Autodesk Inventor part; units mm, degrees
(part 4 of 5)
  line L2308 (121.595, 74.0625) -> (121.595, 60.2629) projected
  line L2309 (121.595, 74.0625) -> (121.595, 60.2629) projected
  line L2310 (121.595, 60.2629) -> (107.794, 60.2629) projected
  line L2311 (121.595, 60.2629) -> (107.794, 60.2629) projected
  line L2312 (121.595, 74.0625) -> (121.595, 60.2629) projected
  line L2313 (121.595, 74.0625) -> (121.595, 60.2629) projected
  line L2314 (107.794, 74.0625) -> (121.595, 74.0625) projected
  line L2315 (107.794, 74.0625) -> (121.595, 74.0625) projected
  line L2316 (121.595, 60.2629) -> (107.794, 60.2629) projected
  line L2317 (121.595, 60.2629) -> (107.794, 60.2629) projected
  line L2318 (107.794, 60.2629) -> (107.794, 74.0625) projected
  line L2319 (107.794, 60.2629) -> (107.794, 74.0625) projected
  line L2320 (102.545, 74.0625) -> (102.545, 60.2629) projected
  line L2321 (102.545, 74.0625) -> (102.545, 60.2629) projected
  line L2322 (102.545, 60.2629) -> (88.7444, 60.2629) projected
  line L2323 (102.545, 60.2629) -> (88.7444, 60.2629) projected
  line L2324 (88.7444, 60.2629) -> (88.7444, 74.0625) projected
  line L2325 (88.7444, 60.2629) -> (88.7444, 74.0625) projected
  line L2326 (88.7444, 74.0625) -> (102.545, 74.0625) projected
  line L2327 (88.7444, 74.0625) -> (102.545, 74.0625) projected
  line L2328 (88.2579, 55.0125) -> (88.2579, 41.2129) projected
  line L2329 (88.2579, 55.0125) -> (88.2579, 41.2129) projected
  line L2330 (88.2579, 41.2129) -> (74.4583, 41.2129) projected
  line L2331 (88.2579, 41.2129) -> (74.4583, 41.2129) projected
  line L2332 (74.4583, 55.0125) -> (88.2579, 55.0125) projected
  line L2333 (74.4583, 55.0125) -> (88.2579, 55.0125) projected
  line L2334 (74.4583, 41.2129) -> (74.4583, 55.0125) projected
  line L2335 (74.4583, 41.2129) -> (74.4583, 55.0125) projected
  line L2336 (69.2079, 55.0125) -> (69.2079, 41.2129) projected
  line L2337 (69.2079, 55.0125) -> (69.2079, 41.2129) projected
  line L2338 (93.5083, 41.2129) -> (93.5083, 55.0125) projected
  line L2339 (93.5083, 41.2129) -> (93.5083, 55.0125) projected
  line L2340 (112.07, 116.926) -> (112.07, 103.125) projected
  line L2341 (112.07, 103.125) -> (98.2694, 103.125) projected
  line L2342 (112.07, 103.125) -> (98.2694, 103.125) projected
  line L2343 (98.2694, 103.125) -> (98.2694, 116.926) projected
  line L2344 (98.2694, 116.926) -> (112.07, 116.926) projected
  line L2345 (98.2694, 116.926) -> (112.07, 116.926) projected
  line L2346 (112.07, 116.926) -> (112.07, 103.125) projected
  line L2347 (135.883, 116.926) -> (135.883, 103.125) projected
  line L2348 (135.883, 116.926) -> (135.883, 103.125) projected
  line L2349 (135.883, 103.125) -> (122.083, 103.125) projected
  line L2350 (98.2694, 103.125) -> (98.2694, 116.926) projected
  line L2351 (135.883, 103.125) -> (122.083, 103.125) projected
  line L2352 (73.9704, 116.926) -> (73.9704, 103.125) projected
  line L2353 (73.9704, 116.926) -> (73.9704, 103.125) projected
  line L2354 (93.0204, 103.125) -> (79.2194, 103.125) projected
  line L2355 (93.0204, 103.125) -> (79.2194, 103.125) projected
  line L2356 (93.0204, 116.926) -> (93.0204, 103.125) projected
  line L2357 (93.0204, 116.926) -> (93.0204, 103.125) projected
  line L2358 (93.0204, 116.926) -> (93.0204, 103.125) projected
  line L2359 (93.0204, 116.926) -> (93.0204, 103.125) projected
  line L2360 (93.0204, 93.1125) -> (93.0204, 79.3129) projected
  line L2361 (93.0204, 93.1125) -> (93.0204, 79.3129) projected
  line L2362 (79.2194, 79.3129) -> (79.2194, 93.1125) projected
  line L2363 (79.2194, 79.3129) -> (79.2194, 93.1125) projected
  line L2364 (79.2194, 93.1125) -> (93.0204, 93.1125) projected
  line L2365 (79.2194, 93.1125) -> (93.0204, 93.1125) projected
  line L2366 (93.0204, 103.125) -> (79.2194, 103.125) projected
  line L2367 (93.0204, 103.125) -> (79.2194, 103.125) projected
  line L2368 (79.2194, 116.926) -> (93.0204, 116.926) projected
  line L2369 (79.2194, 116.926) -> (93.0204, 116.926) projected
  line L2370 (79.2194, 116.926) -> (93.0204, 116.926) projected
  line L2371 (79.2194, 116.926) -> (93.0204, 116.926) projected
  line L2372 (79.2194, 103.125) -> (79.2194, 116.926) projected
  line L2373 (79.2194, 103.125) -> (79.2194, 116.926) projected
  line L2374 (79.2194, 103.125) -> (79.2194, 116.926) projected
  line L2375 (79.2194, 103.125) -> (79.2194, 116.926) projected
  line L2376 (73.9704, 103.125) -> (60.1694, 103.125) projected
  line L2377 (73.9704, 103.125) -> (60.1694, 103.125) projected
  line L2378 (60.1694, 103.125) -> (60.1694, 116.926) projected
  line L2379 (60.1694, 103.125) -> (60.1694, 116.926) projected
  line L2380 (60.1694, 116.926) -> (73.9704, 116.926) projected
  line L2381 (60.1694, 116.926) -> (73.9704, 116.926) projected
  line L2382 (54.919, 103.125) -> (41.1208, 103.125) projected
  line L2383 (54.919, 103.125) -> (41.1208, 103.125) projected
  line L2384 (41.1208, 103.125) -> (41.1208, 116.926) projected
  line L2385 (41.1208, 103.125) -> (41.1208, 116.926) projected
  line L2386 (41.1208, 116.926) -> (54.919, 116.926) projected
  line L2387 (41.1208, 116.926) -> (54.919, 116.926) projected
  line L2388 (54.919, 116.926) -> (54.919, 103.125) projected
  line L2389 (73.9704, 103.125) -> (60.1694, 103.125) projected
  line L2390 (73.9704, 103.125) -> (60.1694, 103.125) projected
  line L2391 (60.1694, 116.926) -> (73.9704, 116.926) projected
  line L2392 (60.1694, 116.926) -> (73.9704, 116.926) projected
  line L2393 (73.9704, 116.926) -> (73.9704, 103.125) projected
  line L2394 (73.9704, 116.926) -> (73.9704, 103.125) projected
  line L2395 (41.1208, 93.1125) -> (54.919, 93.1125) projected
  line L2396 (41.1208, 93.1125) -> (54.919, 93.1125) projected
  line L2397 (41.1208, 93.1125) -> (54.919, 93.1125) projected
  line L2398 (60.1694, 103.125) -> (60.1694, 116.926) projected
  line L2399 (60.1694, 103.125) -> (60.1694, 116.926) projected
  line L2400 (54.919, 103.125) -> (41.1208, 103.125) projected
  line L2401 (54.919, 103.125) -> (41.1208, 103.125) projected
  line L2402 (54.919, 116.926) -> (54.919, 103.125) projected
  line L2403 (54.919, 116.926) -> (54.919, 103.125) projected
  line L2404 (54.919, 116.926) -> (54.919, 103.125) projected
  line L2405 (41.1208, 116.926) -> (54.919, 116.926) projected
  line L2406 (41.1208, 116.926) -> (54.919, 116.926) projected
  line L2407 (41.1208, 93.1125) -> (54.919, 93.1125) projected
  line L2408 (88.7444, 60.2629) -> (88.7444, 74.0625) projected
  line L2409 (88.7444, 60.2629) -> (88.7444, 74.0625) projected
  line L2410 (79.2194, 79.3129) -> (79.2194, 93.1125) projected
  line L2411 (79.2194, 79.3129) -> (79.2194, 93.1125) projected
  line L2412 (79.2194, 93.1125) -> (93.0204, 93.1125) projected
  line L2413 (79.2194, 93.1125) -> (93.0204, 93.1125) projected
  line L2414 (93.0204, 93.1125) -> (93.0204, 79.3129) projected
  line L2415 (93.0204, 93.1125) -> (93.0204, 79.3129) projected
  line L2416 (93.0204, 79.3129) -> (79.2194, 79.3129) projected
  line L2417 (93.0204, 79.3129) -> (79.2194, 79.3129) projected
  line L2418 (83.4954, 60.2629) -> (69.6958, 60.2629) projected
  line L2419 (69.6958, 74.0625) -> (83.4954, 74.0625) projected
  line L2420 (69.6958, 74.0625) -> (83.4954, 74.0625) projected
  line L2421 (83.4954, 74.0625) -> (83.4954, 60.2629) projected
  line L2422 (83.4954, 74.0625) -> (83.4954, 60.2629) projected
  line L2423 (83.4954, 60.2629) -> (69.6958, 60.2629) projected
  line L2424 (83.4954, 60.2629) -> (69.6958, 60.2629) projected
  line L2425 (83.4954, 74.0625) -> (83.4954, 60.2629) projected
  line L2426 (83.4954, 74.0625) -> (83.4954, 60.2629) projected
  line L2427 (69.6958, 74.0625) -> (83.4954, 74.0625) projected
  line L2428 (69.6958, 74.0625) -> (83.4954, 74.0625) projected
  line L2429 (93.0204, 79.3129) -> (79.2194, 79.3129) projected
  line L2430 (93.0204, 79.3129) -> (79.2194, 79.3129) projected
  line L2431 (83.4954, 60.2629) -> (69.6958, 60.2629) projected
  line L2432 (41.1208, 79.3129) -> (41.1208, 93.1125) projected
  line L2433 (41.1208, 79.3129) -> (41.1208, 93.1125) projected
  line L2434 (16.8203, 103.125) -> (3.0193, 103.125) projected
  line L2435 (16.8203, 103.125) -> (3.0193, 103.125) projected
  line L2436 (3.0193, 103.125) -> (3.0193, 116.926) projected
  line L2437 (3.0193, 103.125) -> (3.0193, 116.926) projected
  line L2438 (3.0193, 116.926) -> (16.8203, 116.926) projected
  line L2439 (3.0193, 116.926) -> (16.8203, 116.926) projected
  line L2440 (3.0193, 79.3129) -> (3.0193, 93.1125) projected
  line L2441 (3.0193, 93.1125) -> (16.8203, 93.1125) projected
  line L2442 (3.0193, 93.1125) -> (16.8203, 93.1125) projected
  line L2443 (16.8203, 93.1125) -> (16.8203, 79.3129) projected
  line L2444 (16.8203, 93.1125) -> (16.8203, 79.3129) projected
  line L2445 (16.8203, 93.1125) -> (16.8203, 79.3129) projected
  line L2446 (16.8203, 93.1125) -> (16.8203, 79.3129) projected
  line L2447 (3.0193, 93.1125) -> (16.8203, 93.1125) projected
  line L2448 (3.0193, 93.1125) -> (16.8203, 93.1125) projected
  line L2449 (3.0193, 79.3129) -> (3.0193, 93.1125) projected
  line L2450 (3.0193, 79.3129) -> (3.0193, 93.1125) projected
  line L2451 (22.0707, 79.3129) -> (22.0707, 93.1125) projected
  line L2452 (22.0707, 79.3129) -> (22.0707, 93.1125) projected
  line L2453 (0.0951, 117.85) -> (0.0951, 2.1869) projected
  line L2454 (0.0951, 117.85) -> (0.0951, 2.187) projected
  line L2455 (41.1208, 103.125) -> (41.1208, 116.926) projected
  line L2456 (41.1208, 103.125) -> (41.1208, 116.926) projected
  line L2457 (16.8203, 116.926) -> (16.8203, 103.125) projected
  line L2458 (16.8203, 116.926) -> (16.8203, 103.125) projected
  line L2459 (3.0193, 79.3129) -> (3.0193, 93.1125) projected
  line L2460 (22.0707, 79.3129) -> (22.0707, 93.1125) projected
  line L2461 (22.0707, 79.3129) -> (22.0707, 93.1125) projected
  line L2462 (35.8704, 79.3129) -> (22.0707, 79.3129) projected
  line L2463 (35.8704, 79.3129) -> (22.0707, 79.3129) projected
  line L2464 (35.8704, 79.3129) -> (22.0707, 79.3129) projected
  line L2465 (22.0707, 93.1125) -> (35.8704, 93.1125) projected
  line L2466 (22.0707, 93.1125) -> (35.8704, 93.1125) projected
  line L2467 (22.0707, 93.1125) -> (35.8704, 93.1125) projected
  line L2468 (35.8704, 79.3129) -> (22.0707, 79.3129) projected
  line L2469 (22.0707, 93.1125) -> (35.8704, 93.1125) projected
  line L2470 (35.8704, 93.1125) -> (35.8704, 79.3129) projected
  line L2471 (35.8704, 93.1125) -> (35.8704, 79.3129) projected
  line L2472 (35.8704, 93.1125) -> (35.8704, 79.3129) projected
  line L2473 (35.8704, 93.1125) -> (35.8704, 79.3129) projected
  line L2474 (31.5957, 60.2629) -> (31.5957, 74.0625) projected
  line L2475 (31.5957, 60.2629) -> (31.5957, 74.0625) projected
  line L2476 (31.5957, 60.2629) -> (31.5957, 74.0625) projected
  line L2477 (31.5957, 74.0625) -> (45.3954, 74.0625) projected
  line L2478 (31.5957, 74.0625) -> (45.3954, 74.0625) projected
  line L2479 (31.5957, 74.0625) -> (45.3954, 74.0625) projected
  line L2480 (31.5957, 74.0625) -> (45.3954, 74.0625) projected
  line L2481 (31.5957, 60.2629) -> (31.5957, 74.0625) projected
  line L2482 (16.8203, 79.3129) -> (3.0193, 79.3129) projected
  line L2483 (16.8203, 79.3129) -> (3.0193, 79.3129) projected
  line L2484 (7.7832, 74.0625) -> (21.5828, 74.0625) projected
  line L2485 (7.7832, 74.0625) -> (21.5828, 74.0625) projected
  line L2486 (21.5828, 74.0625) -> (21.5828, 60.2629) projected
  line L2487 (21.5828, 74.0625) -> (21.5828, 60.2629) projected
  line L2488 (7.7832, 60.2629) -> (7.7832, 74.0625) projected
  line L2489 (7.7832, 60.2629) -> (7.7832, 74.0625) projected
  line L2490 (7.7832, 60.2629) -> (7.7832, 74.0625) projected
  line L2491 (7.7832, 60.2629) -> (7.7832, 74.0625) projected
  line L2492 (21.5828, 74.0625) -> (21.5828, 60.2629) projected
  line L2493 (21.5828, 74.0625) -> (21.5828, 60.2629) projected
  line L2494 (16.8203, 79.3129) -> (3.0193, 79.3129) projected
  line L2495 (16.8203, 79.3129) -> (3.0193, 79.3129) projected
  line L2496 (21.5828, 60.2629) -> (7.7832, 60.2629) projected
  line L2497 (21.5828, 60.2629) -> (7.7832, 60.2629) projected
  line L2498 (21.5828, 60.2629) -> (7.7832, 60.2629) projected
  line L2499 (21.5828, 60.2629) -> (7.7832, 60.2629) projected
  line L2500 (10.163, 55.0125) -> (23.9641, 55.0125) projected
  line L2501 (10.163, 55.0125) -> (23.9641, 55.0125) projected
  line L2502 (10.163, 55.0125) -> (23.9641, 55.0125) projected
  line L2503 (10.163, 55.0125) -> (23.9641, 55.0125) projected
  line L2504 (23.9641, 55.0125) -> (23.9641, 41.2129) projected
  line L2505 (23.9641, 55.0125) -> (23.9641, 41.2129) projected
  line L2506 (23.9641, 55.0125) -> (23.9641, 41.2129) projected
  line L2507 (23.9641, 55.0125) -> (23.9641, 41.2129) projected
  line L2508 (10.163, 41.2129) -> (10.163, 55.0125) projected
  line L2509 (10.163, 41.2129) -> (10.163, 55.0125) projected
  line L2510 (10.163, 41.2129) -> (10.163, 55.0125) projected
  line L2511 (10.163, 41.2129) -> (10.163, 55.0125) projected
  line L2512 (23.9641, 41.2129) -> (10.163, 41.2129) projected
  line L2513 (23.9641, 41.2129) -> (10.163, 41.2129) projected
  line L2514 (23.9641, 41.2129) -> (10.163, 41.2129) projected
  line L2515 (23.9641, 41.2129) -> (10.163, 41.2129) projected
  line L2516 (45.3954, 60.2629) -> (31.5957, 60.2629) projected
  line L2517 (45.3954, 60.2629) -> (31.5957, 60.2629) projected
  line L2518 (50.1579, 55.0125) -> (50.1579, 41.2129) projected
  line L2519 (50.1579, 55.0125) -> (50.1579, 41.2129) projected
  line L2520 (45.8833, 35.9625) -> (59.6829, 35.9625) projected
  line L2521 (45.8833, 35.9625) -> (59.6829, 35.9625) projected
  line L2522 (50.1579, 55.0125) -> (50.1579, 41.2129) projected
  line L2523 (50.1579, 55.0125) -> (50.1579, 41.2129) projected
  line L2524 (37.0018, 31.2636) -> (37.8273, 31.2636) projected
  line L2525 (37.0018, 31.2636) -> (37.8273, 31.2636) projected
  line L2526 (37.0018, 34.4923) -> (37.0018, 31.2636) projected
  line L2527 (37.0018, 34.4923) -> (37.0018, 31.2636) projected
  line L2528 (50.1579, 41.2129) -> (36.3583, 41.2129) projected
  line L2529 (50.1579, 41.2129) -> (36.3583, 41.2129) projected
  line L2530 (50.1579, 41.2129) -> (36.3583, 41.2129) projected
  line L2531 (50.1579, 41.2129) -> (36.3583, 41.2129) projected
  line L2532 (36.3583, 55.0125) -> (50.1579, 55.0125) projected
  line L2533 (36.3583, 55.0125) -> (50.1579, 55.0125) projected
  line L2534 (36.3583, 55.0125) -> (50.1579, 55.0125) projected
  line L2535 (36.3583, 55.0125) -> (50.1579, 55.0125) projected
  line L2536 (36.3583, 41.2129) -> (36.3583, 55.0125) projected
  line L2537 (36.3583, 41.2129) -> (36.3583, 55.0125) projected
  line L2538 (36.3583, 41.2129) -> (36.3583, 55.0125) projected
  line L2539 (36.3583, 41.2129) -> (36.3583, 55.0125) projected
  line L2540 (45.3954, 60.2629) -> (31.5957, 60.2629) projected
  line L2541 (45.3954, 60.2629) -> (31.5957, 60.2629) projected
  line L2542 (84.6391, 7.8135) -> (84.6391, 3.3431) projected
  line L2543 (84.6391, 7.8135) -> (84.6391, 3.3431) projected
  line L2544 (84.6391, 3.3431) -> (82.9137, 3.3431) projected
  line L2545 (84.6391, 3.3431) -> (82.9137, 3.3431) projected
  line L2546 (82.9137, 3.3431) -> (82.9137, 2.1429) projected
  line L2547 (82.9137, 3.3431) -> (82.9137, 2.1429) projected
  line L2548 (82.9137, 2.1429) -> (79.8132, 2.1429) projected
  line L2549 (82.9137, 2.1429) -> (79.8132, 2.1429) projected
  line L2550 (79.8132, 2.1429) -> (79.8132, 3.3431) projected
  line L2551 (78.0881, 3.3431) -> (78.0881, 9.6132) projected
  line L2552 (78.0881, 3.3431) -> (78.0881, 9.6132) projected
  line L2553 (78.0881, 3.3431) -> (78.0881, 9.6132) projected
  line L2554 (78.0881, 3.3431) -> (78.0881, 9.6132) projected
  line L2555 (84.6391, 7.8135) -> (84.6391, 3.3431) projected
  line L2556 (84.6391, 7.8135) -> (84.6391, 3.3431) projected
  line L2557 (84.6391, 3.3431) -> (82.9137, 3.3431) projected
  line L2558 (84.6391, 3.3431) -> (82.9137, 3.3431) projected
  line L2559 (79.8132, 3.3431) -> (78.0881, 3.3431) projected
  line L2560 (79.8132, 3.3431) -> (78.0881, 3.3431) projected
  line L2561 (79.8132, 3.3431) -> (78.0881, 3.3431) projected
  line L2562 (79.8132, 3.3431) -> (78.0881, 3.3431) projected
  line L2563 (79.8132, 2.1429) -> (79.8132, 3.3431) projected
  line L2564 (79.8132, 2.1429) -> (79.8132, 3.3431) projected
  line L2565 (79.8132, 2.1429) -> (79.8132, 3.3431) projected
  line L2566 (82.9137, 3.3431) -> (82.9137, 2.1429) projected
  line L2567 (82.9137, 3.3431) -> (82.9137, 2.1429) projected
  line L2568 (82.9137, 2.1429) -> (79.8132, 2.1429) projected
  line L2569 (82.9137, 2.1429) -> (79.8132, 2.1429) projected
  line L2570 (28.7266, 35.9625) -> (28.7266, 31.2636) projected
  line L2571 (28.7266, 35.9625) -> (28.7266, 31.2636) projected
  line L2572 (28.7266, 31.2636) -> (30.4519, 31.2636) projected
  line L2573 (28.7266, 26.8635) -> (28.7266, 22.163) projected
  line L2574 (28.7266, 26.8635) -> (28.7266, 22.163) projected
  line L2575 (30.4519, 26.8635) -> (28.7266, 26.8635) projected
  line L2576 (30.4519, 26.8635) -> (28.7266, 26.8635) projected
  line L2577 (30.4519, 26.8635) -> (28.7266, 26.8635) projected
  line L2578 (30.4519, 26.8635) -> (28.7266, 26.8635) projected
  line L2579 (30.4519, 22.3931) -> (30.4519, 26.8635) projected
  line L2580 (30.4519, 22.3931) -> (30.4519, 26.8635) projected
  line L2581 (32.1758, 21.1928) -> (32.1758, 22.3931) projected
  line L2582 (32.1758, 21.1928) -> (32.1758, 22.3931) projected
  line L2583 (32.1758, 22.3931) -> (30.4519, 22.3931) projected
  line L2584 (32.1758, 22.3931) -> (30.4519, 22.3931) projected
  line L2585 (28.7266, 31.2636) -> (30.4519, 31.2636) projected
  line L2586 (28.7266, 31.2636) -> (30.4519, 31.2636) projected
  line L2587 (28.7266, 31.2636) -> (30.4519, 31.2636) projected
  line L2588 (28.7266, 35.9625) -> (28.7266, 31.2636) projected
  line L2589 (28.7266, 35.9625) -> (28.7266, 31.2636) projected
  line L2590 (30.4519, 31.2636) -> (30.4519, 34.4923) projected
  line L2591 (30.4519, 31.2636) -> (30.4519, 34.4923) projected
  line L2592 (30.4519, 31.2636) -> (30.4519, 34.4923) projected
  line L2593 (30.4519, 31.2636) -> (30.4519, 34.4923) projected
  line L2594 (30.4519, 34.4923) -> (37.0018, 34.4923) projected
  line L2595 (30.4519, 34.4923) -> (37.0018, 34.4923) projected
  line L2596 (30.4519, 34.4923) -> (37.0018, 34.4923) projected
  line L2597 (30.4519, 34.4923) -> (37.0018, 34.4923) projected
  line L2598 (28.7266, 26.8635) -> (28.7266, 22.163) projected
  line L2599 (28.7266, 26.8635) -> (28.7266, 22.163) projected
  line L2600 (14.9269, 31.2636) -> (14.9269, 35.9625) projected
  line L2601 (14.9269, 31.2636) -> (14.9269, 35.9625) projected
  line L2602 (14.9269, 31.2636) -> (14.9269, 35.9625) projected
  line L2603 (14.9269, 31.2636) -> (14.9269, 35.9625) projected
  line L2604 (37.0018, 34.4923) -> (37.0018, 31.2636) projected
  line L2605 (37.0018, 34.4923) -> (37.0018, 31.2636) projected
  line L2606 (37.0018, 28.6632) -> (37.0018, 22.3931) projected
  line L2607 (37.0018, 28.6632) -> (37.0018, 22.3931) projected
  line L2608 (37.0018, 28.6632) -> (37.0018, 22.3931) projected
  line L2609 (37.0018, 28.6632) -> (37.0018, 22.3931) projected
  line L2610 (37.8273, 28.6632) -> (37.0018, 28.6632) projected
  line L2611 (37.8273, 28.6632) -> (37.0018, 28.6632) projected
  line L2612 (37.8273, 28.6632) -> (37.0018, 28.6632) projected
  line L2613 (37.8273, 28.6632) -> (37.0018, 28.6632) projected
  line L2614 (37.0018, 31.2636) -> (37.8273, 31.2636) projected
  line L2615 (37.0018, 31.2636) -> (37.8273, 31.2636) projected
  line L2616 (37.8273, 31.2636) -> (37.8273, 28.6632) projected
  line L2617 (37.8273, 31.2636) -> (37.8273, 28.6632) projected
  line L2618 (45.8833, 22.163) -> (45.8833, 35.9625) projected
  line L2619 (45.8833, 22.163) -> (45.8833, 35.9625) projected
  line L2620 (59.6829, 22.163) -> (45.8833, 22.163) projected
  line L2621 (59.6829, 22.163) -> (45.8833, 22.163) projected
  line L2622 (59.6829, 35.9625) -> (59.6829, 22.163) projected
  line L2623 (59.6829, 35.9625) -> (59.6829, 22.163) projected
  line L2624 (37.8273, 31.2636) -> (37.8273, 28.6632) projected
  line L2625 (37.8273, 31.2636) -> (37.8273, 28.6632) projected
  line L2626 (32.1758, 22.3931) -> (30.4519, 22.3931) projected
  line L2627 (32.1758, 22.3931) -> (30.4519, 22.3931) projected
  line L2628 (30.4519, 22.3931) -> (30.4519, 26.8635) projected
  line L2629 (30.4519, 22.3931) -> (30.4519, 26.8635) projected
  line L2630 (37.0018, 22.3931) -> (35.2764, 22.3931) projected
  line L2631 (37.0018, 22.3931) -> (35.2764, 22.3931) projected
  line L2632 (37.0018, 22.3931) -> (35.2764, 22.3931) projected
  line L2633 (37.0018, 22.3931) -> (35.2764, 22.3931) projected
  line L2634 (35.2764, 22.3931) -> (35.2764, 21.1928) projected
  line L2635 (35.2764, 22.3931) -> (35.2764, 21.1928) projected
  line L2636 (35.2764, 22.3931) -> (35.2764, 21.1928) projected
  line L2637 (35.2764, 22.3931) -> (35.2764, 21.1928) projected
  line L2638 (35.2764, 21.1928) -> (32.1758, 21.1928) projected
  line L2639 (35.2764, 21.1928) -> (32.1758, 21.1928) projected
  line L2640 (35.2764, 21.1928) -> (32.1758, 21.1928) projected
  line L2641 (35.2764, 21.1928) -> (32.1758, 21.1928) projected
  line L2642 (32.1758, 21.1928) -> (32.1758, 22.3931) projected
  line L2643 (32.1758, 21.1928) -> (32.1758, 22.3931) projected
  line L2644 (29.213, 16.9127) -> (43.0142, 16.9127) projected
  line L2645 (29.213, 16.9127) -> (43.0142, 16.9127) projected
  line L2646 (43.0142, 16.9127) -> (43.0142, 3.113) projected
  line L2647 (43.0142, 16.9127) -> (43.0142, 3.113) projected
  line L2648 (29.213, 3.113) -> (29.213, 16.9127) projected
  line L2649 (29.213, 3.113) -> (29.213, 16.9127) projected
  line L2650 (43.0142, 3.113) -> (29.213, 3.113) projected
  line L2651 (43.0142, 3.113) -> (29.213, 3.113) projected
  line L2652 (74.4583, 41.2129) -> (74.4583, 55.0125) projected
  line L2653 (74.4583, 41.2129) -> (74.4583, 55.0125) projected
  line L2654 (74.4583, 55.0125) -> (88.2579, 55.0125) projected
  line L2655 (74.4583, 55.0125) -> (88.2579, 55.0125) projected
  line L2656 (88.2579, 55.0125) -> (88.2579, 41.2129) projected
  line L2657 (88.2579, 55.0125) -> (88.2579, 41.2129) projected
  line L2658 (88.2579, 41.2129) -> (74.4583, 41.2129) projected
  line L2659 (88.2579, 41.2129) -> (74.4583, 41.2129) projected
  line L2660 (83.9833, 22.163) -> (83.9833, 35.9625) projected
  line L2661 (83.9833, 22.163) -> (83.9833, 35.9625) projected
  line L2662 (78.7329, 22.163) -> (64.9333, 22.163) projected
  line L2663 (78.7329, 22.163) -> (64.9333, 22.163) projected
  line L2664 (64.9333, 22.163) -> (64.9333, 35.9625) projected
  line L2665 (64.9333, 22.163) -> (64.9333, 35.9625) projected
  line L2666 (64.9333, 35.9625) -> (78.7329, 35.9625) projected
  line L2667 (64.9333, 35.9625) -> (78.7329, 35.9625) projected
  line L2668 (78.7329, 35.9625) -> (78.7329, 22.163) projected
  line L2669 (78.7329, 35.9625) -> (78.7329, 22.163) projected
  line L2670 (78.7329, 22.163) -> (64.9333, 22.163) projected
  line L2671 (78.7329, 22.163) -> (64.9333, 22.163) projected
  line L2672 (64.9333, 35.9625) -> (78.7329, 35.9625) projected
  line L2673 (64.9333, 35.9625) -> (78.7329, 35.9625) projected
  line L2674 (64.9333, 22.163) -> (64.9333, 35.9625) projected
  line L2675 (64.9333, 22.163) -> (64.9333, 35.9625) projected
  line L2676 (55.4083, 41.2129) -> (55.4083, 55.0125) projected
  line L2677 (55.4083, 41.2129) -> (55.4083, 55.0125) projected
  line L2678 (55.4083, 41.2129) -> (55.4083, 55.0125) projected
  line L2679 (55.4083, 41.2129) -> (55.4083, 55.0125) projected
  line L2680 (55.4083, 55.0125) -> (69.2079, 55.0125) projected
  line L2681 (55.4083, 55.0125) -> (69.2079, 55.0125) projected
  line L2682 (69.2079, 55.0125) -> (69.2079, 41.2129) projected
  line L2683 (69.2079, 55.0125) -> (69.2079, 41.2129) projected
  line L2684 (55.4083, 55.0125) -> (69.2079, 55.0125) projected
  line L2685 (55.4083, 55.0125) -> (69.2079, 55.0125) projected
  line L2686 (69.2079, 41.2129) -> (55.4083, 41.2129) projected
  line L2687 (69.2079, 41.2129) -> (55.4083, 41.2129) projected
  line L2688 (69.2079, 41.2129) -> (55.4083, 41.2129) projected
  line L2689 (69.2079, 41.2129) -> (55.4083, 41.2129) projected
  line L2690 (13.2016, 31.2636) -> (14.9269, 31.2636) projected
  line L2691 (13.2016, 31.2636) -> (14.9269, 31.2636) projected
  line L2692 (13.2016, 31.2636) -> (14.9269, 31.2636) projected
  line L2693 (13.2016, 31.2636) -> (14.9269, 31.2636) projected
  line L2694 (5.8263, 28.6632) -> (5.8263, 31.2636) projected
  line L2695 (5.8263, 28.6632) -> (5.8263, 31.2636) projected
  line L2696 (5.8263, 28.6632) -> (5.8263, 31.2636) projected
  line L2697 (5.8263, 28.6632) -> (5.8263, 31.2636) projected
  line L2698 (5.8263, 31.2636) -> (6.6518, 31.2636) projected
  line L2699 (5.8263, 31.2636) -> (6.6518, 31.2636) projected
  line L2700 (5.8263, 31.2636) -> (6.6518, 31.2636) projected
  line L2701 (6.6518, 34.4923) -> (13.2016, 34.4923) projected
  line L2702 (13.2016, 34.4923) -> (13.2016, 31.2636) projected
  line L2703 (13.2016, 34.4923) -> (13.2016, 31.2636) projected
  line L2704 (13.2016, 34.4923) -> (13.2016, 31.2636) projected
  line L2705 (6.6518, 34.4923) -> (13.2016, 34.4923) projected
  line L2706 (6.6518, 34.4923) -> (13.2016, 34.4923) projected
  line L2707 (6.6518, 34.4923) -> (13.2016, 34.4923) projected
  line L2708 (13.2016, 34.4923) -> (13.2016, 31.2636) projected
  line L2709 (6.6518, 31.2636) -> (6.6518, 34.4923) projected
  line L2710 (6.6518, 31.2636) -> (6.6518, 34.4923) projected
  line L2711 (6.6518, 31.2636) -> (6.6518, 34.4923) projected
  line L2712 (6.6518, 31.2636) -> (6.6518, 34.4923) projected
  line L2713 (5.8263, 31.2636) -> (6.6518, 31.2636) projected
  line L2714 (13.2016, 22.3931) -> (11.4763, 22.3931) projected
  line L2715 (13.2016, 22.3931) -> (11.4763, 22.3931) projected
  line L2716 (11.4763, 22.3931) -> (11.4763, 21.1928) projected
  line L2717 (11.4763, 22.3931) -> (11.4763, 21.1928) projected
  line L2718 (11.4763, 21.1928) -> (8.3771, 21.1928) projected
  line L2719 (11.4763, 21.1928) -> (8.3771, 21.1928) projected
  line L2720 (8.3771, 21.1928) -> (8.3771, 22.3931) projected
  line L2721 (8.3771, 21.1928) -> (8.3771, 22.3931) projected
  line L2722 (8.3771, 22.3931) -> (6.6518, 22.3931) projected
  line L2723 (8.3771, 22.3931) -> (6.6518, 22.3931) projected
  line L2724 (11.4763, 22.3931) -> (11.4763, 21.1928) projected
  line L2725 (11.4763, 22.3931) -> (11.4763, 21.1928) projected
  line L2726 (11.4763, 21.1928) -> (8.3771, 21.1928) projected
  line L2727 (11.4763, 21.1928) -> (8.3771, 21.1928) projected
  line L2728 (8.3771, 21.1928) -> (8.3771, 22.3931) projected
  line L2729 (8.3771, 21.1928) -> (8.3771, 22.3931) projected
  line L2730 (5.4019, 16.9127) -> (19.2016, 16.9127) projected
  line L2731 (5.4019, 16.9127) -> (19.2016, 16.9127) projected
  line L2732 (5.4019, 3.113) -> (5.4019, 16.9127) projected
  line L2733 (5.4019, 3.113) -> (5.4019, 16.9127) projected
  line L2734 (19.2016, 3.113) -> (5.4019, 3.113) projected
  line L2735 (19.2016, 3.113) -> (5.4019, 3.113) projected
  line L2736 (19.2016, 16.9127) -> (19.2016, 3.113) projected
  line L2737 (19.2016, 16.9127) -> (19.2016, 3.113) projected
  line L2738 (13.2016, 22.3931) -> (11.4763, 22.3931) projected
  line L2739 (13.2016, 22.3931) -> (11.4763, 22.3931) projected
  line L2740 (78.0881, 15.4423) -> (84.6391, 15.4423) projected
  line L2741 (78.0881, 15.4423) -> (84.6391, 15.4423) projected
  line L2742 (84.6391, 15.4423) -> (84.6391, 12.2136) projected
  line L2743 (84.6391, 15.4423) -> (84.6391, 12.2136) projected
  line L2744 (78.0881, 9.6132) -> (77.264, 9.6132) projected
  line L2745 (78.0881, 9.6132) -> (77.264, 9.6132) projected
  line L2746 (78.0881, 9.6132) -> (77.264, 9.6132) projected
  line L2747 (78.0881, 9.6132) -> (77.264, 9.6132) projected
  line L2748 (77.264, 12.2136) -> (78.0881, 12.2136) projected
  line L2749 (77.264, 9.6132) -> (77.264, 12.2136) projected
  line L2750 (77.264, 9.6132) -> (77.264, 12.2136) projected
  line L2751 (77.264, 9.6132) -> (77.264, 12.2136) projected
  line L2752 (77.264, 12.2136) -> (78.0881, 12.2136) projected
  line L2753 (77.264, 12.2136) -> (78.0881, 12.2136) projected
  line L2754 (77.264, 12.2136) -> (78.0881, 12.2136) projected
  line L2755 (84.6391, 15.4423) -> (84.6391, 12.2136) projected
  line L2756 (84.6391, 15.4423) -> (84.6391, 12.2136) projected
  line L2757 (78.0881, 15.4423) -> (84.6391, 15.4423) projected
  line L2758 (78.0881, 15.4423) -> (84.6391, 15.4423) projected
  line L2759 (78.0881, 12.2136) -> (78.0881, 15.4423) projected
  line L2760 (78.0881, 12.2136) -> (78.0881, 15.4423) projected
  line L2761 (78.0881, 12.2136) -> (78.0881, 15.4423) projected
  line L2762 (78.0881, 12.2136) -> (78.0881, 15.4423) projected
  line L2763 (77.264, 9.6132) -> (77.264, 12.2136) projected
  line L2764 (69.6958, 60.2629) -> (69.6958, 74.0625) projected
  line L2765 (69.6958, 60.2629) -> (69.6958, 74.0625) projected
  line L2766 (64.4454, 74.0625) -> (64.4454, 60.2629) projected
  line L2767 (64.4454, 74.0625) -> (64.4454, 60.2629) projected
  line L2768 (64.4454, 74.0625) -> (64.4454, 60.2629) projected
  line L2769 (64.4454, 74.0625) -> (64.4454, 60.2629) projected
  line L2770 (64.4454, 60.2629) -> (50.6458, 60.2629) projected
  line L2771 (64.4454, 60.2629) -> (50.6458, 60.2629) projected
  line L2772 (64.4454, 60.2629) -> (50.6458, 60.2629) projected
  line L2773 (64.4454, 60.2629) -> (50.6458, 60.2629) projected
  line L2774 (50.6458, 74.0625) -> (64.4454, 74.0625) projected
  line L2775 (50.6458, 60.2629) -> (50.6458, 74.0625) projected
  line L2776 (50.6458, 74.0625) -> (64.4454, 74.0625) projected
  line L2777 (50.6458, 60.2629) -> (50.6458, 74.0625) projected
  line L2778 (50.6458, 60.2629) -> (50.6458, 74.0625) projected
  line L2779 (50.6458, 60.2629) -> (50.6458, 74.0625) projected
  line L2780 (50.6458, 74.0625) -> (64.4454, 74.0625) projected
  line L2781 (50.6458, 74.0625) -> (64.4454, 74.0625) projected
  line L2782 (69.6958, 60.2629) -> (69.6958, 74.0625) projected
  line L2783 (69.6958, 60.2629) -> (69.6958, 74.0625) projected
  line L2784 (53.0271, 16.9127) -> (66.8267, 16.9127) projected
  line L2785 (53.0271, 16.9127) -> (66.8267, 16.9127) projected
  line L2786 (66.8267, 16.9127) -> (66.8267, 3.113) projected
  line L2787 (66.8267, 16.9127) -> (66.8267, 3.113) projected
  line L2788 (66.8267, 3.113) -> (53.0271, 3.113) projected
  line L2789 (66.8267, 3.113) -> (53.0271, 3.113) projected
  line L2790 (53.0271, 3.113) -> (53.0271, 16.9127) projected
  line L2791 (53.0271, 3.113) -> (53.0271, 16.9127) projected
  line L2792 (53.0271, 3.113) -> (53.0271, 16.9127) projected
  line L2793 (53.0271, 3.113) -> (53.0271, 16.9127) projected
  line L2794 (53.0271, 16.9127) -> (66.8267, 16.9127) projected
  line L2795 (53.0271, 16.9127) -> (66.8267, 16.9127) projected
  line L2796 (66.8267, 16.9127) -> (66.8267, 3.113) projected
  line L2797 (66.8267, 16.9127) -> (66.8267, 3.113) projected
  line L2798 (66.8267, 3.113) -> (53.0271, 3.113) projected
  line L2799 (66.8267, 3.113) -> (53.0271, 3.113) projected
  line L2800 (14.9269, 35.9625) -> (28.7266, 35.9625) projected
  line L2801 (14.9269, 35.9625) -> (28.7266, 35.9625) projected
  line L2802 (14.9269, 35.9625) -> (28.7266, 35.9625) projected
  line L2803 (14.9269, 35.9625) -> (28.7266, 35.9625) projected
  line L2804 (28.7266, 22.163) -> (14.9269, 22.163) projected
  line L2805 (28.7266, 22.163) -> (14.9269, 22.163) projected
  line L2806 (28.7266, 22.163) -> (14.9269, 22.163) projected
  line L2807 (28.7266, 22.163) -> (14.9269, 22.163) projected
  line L2808 (14.9269, 22.163) -> (14.9269, 26.8635) projected
  line L2809 (14.9269, 22.163) -> (14.9269, 26.8635) projected
  line L2810 (14.9269, 22.163) -> (14.9269, 26.8635) projected
  line L2811 (14.9269, 22.163) -> (14.9269, 26.8635) projected
  line L2812 (14.9269, 26.8635) -> (13.2016, 26.8635) projected
  line L2813 (14.9269, 26.8635) -> (13.2016, 26.8635) projected
  line L2814 (13.2016, 26.8635) -> (13.2016, 22.3931) projected
  line L2815 (13.2016, 26.8635) -> (13.2016, 22.3931) projected
  line L2816 (6.6518, 22.3931) -> (6.6518, 28.6632) projected
  line L2817 (6.6518, 28.6632) -> (5.8263, 28.6632) projected
  line L2818 (6.6518, 28.6632) -> (5.8263, 28.6632) projected
  line L2819 (6.6518, 28.6632) -> (5.8263, 28.6632) projected
  line L2820 (14.9269, 26.8635) -> (13.2016, 26.8635) projected
  line L2821 (14.9269, 26.8635) -> (13.2016, 26.8635) projected
  line L2822 (6.6518, 22.3931) -> (6.6518, 28.6632) projected
  line L2823 (6.6518, 22.3931) -> (6.6518, 28.6632) projected
  line L2824 (6.6518, 22.3931) -> (6.6518, 28.6632) projected
  line L2825 (8.3771, 22.3931) -> (6.6518, 22.3931) projected
  line L2826 (8.3771, 22.3931) -> (6.6518, 22.3931) projected
  line L2827 (13.2016, 26.8635) -> (13.2016, 22.3931) projected
  line L2828 (13.2016, 26.8635) -> (13.2016, 22.3931) projected
  line L2829 (6.6518, 28.6632) -> (5.8263, 28.6632) projected
  line L2830 (0.0951, 2.1869) -> (0.102, 2.0299) projected
  line L2831 (0.0951, 2.187) -> (0.102, 2.0298) projected
  line L2832 (0.102, 2.0299) -> (0.1199, 1.8741) projected
  line L2833 (0.102, 2.0298) -> (0.1199, 1.8741) projected
  line L2834 (0.1199, 1.8741) -> (0.1502, 1.7198) projected
  line L2835 (0.1199, 1.8741) -> (0.1502, 1.7198) projected
  line L2836 (0.1502, 1.7198) -> (0.1929, 1.5696) projected
  line L2837 (0.1502, 1.7198) -> (0.1929, 1.5696) projected
  line L2838 (0.1929, 1.5696) -> (0.248, 1.4221) projected
  line L2839 (0.1929, 1.5696) -> (0.248, 1.4221) projected
  line L2840 (0.248, 1.4221) -> (0.3128, 1.2788) projected
  line L2841 (0.248, 1.4221) -> (0.3128, 1.2788) projected
  line L2842 (0.3128, 1.2788) -> (0.39, 1.1424) projected
  line L2843 (0.3128, 1.2788) -> (0.39, 1.1424) projected
  line L2844 (0.39, 1.1424) -> (0.4768, 1.0115) projected
  line L2845 (0.39, 1.1424) -> (0.4768, 1.0115) projected
  line L2846 (0.4768, 1.0115) -> (0.5746, 0.8875) projected
  line L2847 (0.4768, 1.0115) -> (0.5746, 0.8875) projected
  line L2848 (0.5746, 0.8875) -> (0.6808, 0.7731) projected
  line L2849 (0.5746, 0.8875) -> (0.6808, 0.7731) projected
  line L2850 (0.6808, 0.7731) -> (0.7965, 0.6656) projected
  line L2851 (0.6808, 0.7731) -> (0.7965, 0.6656) projected
  line L2852 (0.7965, 0.6656) -> (0.9192, 0.5691) projected
  line L2853 (0.7965, 0.6656) -> (0.9192, 0.5691) projected
  line L2854 (1.7818, 0.2122) -> (1.9389, 0.1929) projected
  line L2855 (1.7818, 0.2122) -> (1.9389, 0.1929) projected
  line L2856 (1.6288, 0.2425) -> (1.7818, 0.2122) projected
  line L2857 (1.6288, 0.2425) -> (1.7818, 0.2122) projected
  line L2858 (1.4759, 0.2853) -> (1.6288, 0.2425) projected
  line L2859 (1.4759, 0.2853) -> (1.6288, 0.2425) projected
  line L2860 (1.3298, 0.339) -> (1.4759, 0.2853) projected
  line L2861 (1.3298, 0.339) -> (1.4759, 0.2853) projected
  line L2862 (1.1879, 0.4051) -> (1.3298, 0.339) projected
  line L2863 (1.1879, 0.4051) -> (1.3298, 0.339) projected
  line L2864 (1.0501, 0.4823) -> (1.1879, 0.4051) projected
  line L2865 (1.0501, 0.4823) -> (1.1879, 0.4051) projected
  line L2866 (0.9192, 0.5691) -> (1.0501, 0.4823) projected
  line L2867 (0.9192, 0.5691) -> (1.0501, 0.4823) projected
  line L2868 (1.9389, 0.1929) -> (2.096, 0.1874) projected
  line L2869 (1.9389, 0.1929) -> (2.096, 0.1874) projected
  line L2870 (45.3954, 74.0625) -> (45.3954, 60.2629) projected
  line L2871 (45.3954, 74.0625) -> (45.3954, 60.2629) projected
  line L2872 (45.3954, 74.0625) -> (45.3954, 60.2629) projected
  line L2873 (45.3954, 74.0625) -> (45.3954, 60.2629) projected
  line L2874 (7.7832, 74.0625) -> (21.5828, 74.0625) projected
  line L2875 (7.7832, 74.0625) -> (21.5828, 74.0625) projected
  line L2876 (2.096, 119.849) -> (1.9389, 119.844) projected
  line L2877 (2.096, 119.849) -> (1.9389, 119.844) projected
  line L2878 (1.9389, 119.844) -> (1.7818, 119.826) projected
  line L2879 (1.9389, 119.844) -> (1.7818, 119.826) projected
  line L2880 (1.7818, 119.826) -> (1.6288, 119.796) projected
  line L2881 (1.7818, 119.826) -> (1.6288, 119.796) projected
  line L2882 (1.6288, 119.796) -> (1.4759, 119.753) projected
  line L2883 (1.6288, 119.796) -> (1.4759, 119.753) projected
  line L2884 (1.4759, 119.753) -> (1.3298, 119.698) projected
  line L2885 (1.4759, 119.753) -> (1.3298, 119.698) projected
  line L2886 (1.3298, 119.698) -> (1.1879, 119.633) projected
  line L2887 (1.3298, 119.698) -> (1.1879, 119.633) projected
  line L2888 (1.1879, 119.633) -> (1.0501, 119.556) projected
  line L2889 (1.1879, 119.633) -> (1.0501, 119.556) projected
  line L2890 (1.0501, 119.556) -> (0.9192, 119.469) projected
  line L2891 (1.0501, 119.556) -> (0.9192, 119.469) projected
  line L2892 (0.9192, 119.469) -> (0.7965, 119.371) projected
  line L2893 (0.9192, 119.469) -> (0.7965, 119.371) projected
  line L2894 (0.7965, 119.371) -> (0.6808, 119.265) projected
  line L2895 (0.7965, 119.371) -> (0.6808, 119.265) projected
  line L2896 (0.6808, 119.265) -> (0.5746, 119.149) projected
  line L2897 (0.6808, 119.265) -> (0.5746, 119.149) projected
  line L2898 (16.8203, 103.125) -> (3.0193, 103.125) projected
  line L2899 (16.8203, 103.125) -> (3.0193, 103.125) projected
  line L2900 (16.8203, 116.926) -> (16.8203, 103.125) projected
  line L2901 (16.8203, 116.926) -> (16.8203, 103.125) projected
  line L2902 (3.0193, 116.926) -> (16.8203, 116.926) projected
  line L2903 (3.0193, 116.926) -> (16.8203, 116.926) projected
  line L2904 (3.0193, 103.125) -> (3.0193, 116.926) projected
  line L2905 (3.0193, 103.125) -> (3.0193, 116.926) projected
  line L2906 (0.102, 118.007) -> (0.0951, 117.85) projected
  line L2907 (0.102, 118.007) -> (0.0951, 117.85) projected
  line L2908 (0.1199, 118.163) -> (0.102, 118.007) projected
  line L2909 (0.1199, 118.163) -> (0.102, 118.007) projected
  line L2910 (0.1502, 118.317) -> (0.1199, 118.163) projected
  line L2911 (0.1502, 118.317) -> (0.1199, 118.163) projected
  line L2912 (0.1929, 118.468) -> (0.1502, 118.317) projected
  line L2913 (0.1929, 118.468) -> (0.1502, 118.317) projected
  line L2914 (0.248, 118.616) -> (0.1929, 118.468) projected
  line L2915 (0.248, 118.616) -> (0.1929, 118.468) projected
  line L2916 (0.39, 118.894) -> (0.3128, 118.758) projected
  line L2917 (0.39, 118.894) -> (0.3128, 118.758) projected
  line L2918 (0.4768, 119.025) -> (0.39, 118.894) projected
  line L2919 (0.4768, 119.025) -> (0.39, 118.894) projected
  line L2920 (0.5746, 119.149) -> (0.4768, 119.025) projected
  line L2921 (0.5746, 119.149) -> (0.4768, 119.025) projected
  line L2922 (0.3128, 118.758) -> (0.248, 118.616) projected
  line L2923 (0.3128, 118.758) -> (0.248, 118.616) projected
  line L2924 (54.919, 79.3129) -> (41.1208, 79.3129) projected
  line L2925 (54.919, 79.3129) -> (41.1208, 79.3129) projected
  line L2926 (41.1208, 79.3129) -> (41.1208, 93.1125) projected
  line L2927 (41.1208, 79.3129) -> (41.1208, 93.1125) projected
  line L2928 (54.919, 79.3129) -> (41.1208, 79.3129) projected
  line L2929 (54.919, 79.3129) -> (41.1208, 79.3129) projected
  line L2930 (54.919, 93.1125) -> (54.919, 79.3129) projected
  line L2931 (54.919, 93.1125) -> (54.919, 79.3129) projected
  line L2932 (54.919, 93.1125) -> (54.919, 79.3129) projected
  line L2933 (54.919, 93.1125) -> (54.919, 79.3129) projected
  line L2934 (60.1694, 93.1125) -> (73.9704, 93.1125) projected
  line L2935 (60.1694, 93.1125) -> (73.9704, 93.1125) projected
  line L2936 (60.1694, 79.3129) -> (60.1694, 93.1125) projected
  line L2937 (60.1694, 79.3129) -> (60.1694, 93.1125) projected
  line L2938 (60.1694, 79.3129) -> (60.1694, 93.1125) projected
  line L2939 (60.1694, 79.3129) -> (60.1694, 93.1125) projected
  line L2940 (73.9704, 79.3129) -> (60.1694, 79.3129) projected
  line L2941 (73.9704, 79.3129) -> (60.1694, 79.3129) projected
  line L2942 (73.9704, 93.1125) -> (73.9704, 79.3129) projected
  line L2943 (73.9704, 93.1125) -> (73.9704, 79.3129) projected
  line L2944 (73.9704, 79.3129) -> (60.1694, 79.3129) projected
  line L2945 (73.9704, 79.3129) -> (60.1694, 79.3129) projected
  line L2946 (73.9704, 93.1125) -> (73.9704, 79.3129) projected
  line L2947 (73.9704, 93.1125) -> (73.9704, 79.3129) projected
  line L2948 (60.1694, 93.1125) -> (73.9704, 93.1125) projected
  line L2949 (60.1694, 93.1125) -> (73.9704, 93.1125) projected
  line L2950 (150.658, 55.0125) -> (164.458, 55.0125) projected
  line L2951 (150.658, 55.0125) -> (164.458, 55.0125) projected
  line L2952 (193.033, 103.125) -> (179.233, 103.125) projected
  line L2953 (193.033, 103.125) -> (179.233, 103.125) projected
  line L2954 (179.233, 103.125) -> (179.233, 116.926) projected
  line L2955 (179.233, 103.125) -> (179.233, 116.926) projected
  line L2956 (179.233, 116.926) -> (193.033, 116.926) projected
  line L2957 (179.233, 116.926) -> (193.033, 116.926) projected
  line L2958 (136.371, 79.3129) -> (136.371, 93.1125) projected
  line L2959 (136.371, 79.3129) -> (136.371, 93.1125) projected
  line L2960 (136.371, 93.1125) -> (150.17, 93.1125) projected
  line L2961 (136.371, 93.1125) -> (150.17, 93.1125) projected
  line L2962 (159.695, 74.0625) -> (159.695, 60.2629) projected
  line L2963 (159.695, 74.0625) -> (159.695, 60.2629) projected
  line L2964 (159.695, 60.2629) -> (145.896, 60.2629) projected
  line L2965 (159.695, 60.2629) -> (145.896, 60.2629) projected
  line L2966 (145.896, 74.0625) -> (159.695, 74.0625) projected
  line L2967 (145.896, 74.0625) -> (159.695, 74.0625) projected
  line L2968 (150.17, 93.1125) -> (150.17, 79.3129) projected
  line L2969 (150.17, 93.1125) -> (150.17, 79.3129) projected
  line L2970 (164.946, 60.2629) -> (164.946, 74.0625) projected
  line L2971 (164.946, 60.2629) -> (164.946, 74.0625) projected
  line L2972 (178.745, 74.0625) -> (178.745, 60.2629) projected
  line L2973 (178.745, 74.0625) -> (178.745, 60.2629) projected
  line L2974 (178.745, 60.2629) -> (164.946, 60.2629) projected
  line L2975 (178.745, 60.2629) -> (164.946, 60.2629) projected
  line L2976 (169.708, 55.0125) -> (183.508, 55.0125) projected
  line L2977 (169.708, 55.0125) -> (183.508, 55.0125) projected
  line L2978 (155.421, 79.3129) -> (155.421, 93.1125) projected
  line L2979 (155.421, 79.3129) -> (155.421, 93.1125) projected
  line L2980 (169.22, 79.3129) -> (155.421, 79.3129) projected
  line L2981 (169.22, 79.3129) -> (155.421, 79.3129) projected
  line L2982 (154.933, 103.125) -> (141.133, 103.125) projected
  line L2983 (154.933, 103.125) -> (141.133, 103.125) projected
  line L2984 (164.946, 74.0625) -> (178.745, 74.0625) projected
  line L2985 (164.946, 74.0625) -> (178.745, 74.0625) projected
  line L2986 (169.22, 93.1125) -> (169.22, 79.3129) projected
  line L2987 (169.22, 93.1125) -> (169.22, 79.3129) projected
  line L2988 (155.421, 93.1125) -> (169.22, 93.1125) projected
  line L2989 (155.421, 93.1125) -> (169.22, 93.1125) projected
  line L2990 (141.133, 103.125) -> (141.133, 116.926) projected
  line L2991 (141.133, 103.125) -> (141.133, 116.926) projected
  line L2992 (141.133, 116.926) -> (154.933, 116.926) projected
  line L2993 (141.133, 116.926) -> (154.933, 116.926) projected
  line L2994 (174.471, 79.3129) -> (174.471, 93.1125) projected
  line L2995 (174.471, 79.3129) -> (174.471, 93.1125) projected
  line L2996 (154.933, 116.926) -> (154.933, 103.125) projected
  line L2997 (154.933, 116.926) -> (154.933, 103.125) projected
  line L2998 (173.983, 103.125) -> (160.183, 103.125) projected
  line L2999 (173.983, 103.125) -> (160.183, 103.125) projected
  line L3000 (160.183, 103.125) -> (160.183, 116.926) projected
  line L3001 (160.183, 103.125) -> (160.183, 116.926) projected
  line L3002 (160.183, 116.926) -> (173.983, 116.926) projected
  line L3003 (160.183, 116.926) -> (173.983, 116.926) projected
  line L3004 (173.983, 116.926) -> (173.983, 103.125) projected
  line L3005 (173.983, 116.926) -> (173.983, 103.125) projected
  line L3006 (174.471, 93.1125) -> (188.27, 93.1125) projected
  line L3007 (174.471, 93.1125) -> (188.27, 93.1125) projected
  line L3008 (188.27, 93.1125) -> (188.27, 79.3129) projected
  line L3009 (188.27, 93.1125) -> (188.27, 79.3129) projected
  line L3010 (188.27, 79.3129) -> (174.471, 79.3129) projected
  line L3011 (188.27, 79.3129) -> (174.471, 79.3129) projected
  line L3012 (254.362, 41.4433) -> (254.362, 40.2428) projected
  line L3013 (254.362, 41.4433) -> (254.362, 40.2428) projected
  line L3014 (254.362, 40.2428) -> (251.263, 40.2428) projected
  line L3015 (249.538, 47.7132) -> (248.714, 47.7132) projected
  line L3016 (249.538, 47.7132) -> (248.714, 47.7132) projected
  line L3017 (249.538, 41.4433) -> (249.538, 47.7132) projected
  line L3018 (249.538, 41.4433) -> (249.538, 47.7132) projected
  line L3019 (251.263, 41.4433) -> (249.538, 41.4433) projected
  line L3020 (251.263, 41.4433) -> (249.538, 41.4433) projected
  line L3021 (251.263, 40.2428) -> (251.263, 41.4433) projected
  line L3022 (254.362, 40.2428) -> (251.263, 40.2428) projected
  line L3023 (251.263, 40.2428) -> (251.263, 41.4433) projected
  line L3024 (248.714, 50.3135) -> (249.538, 50.3135) projected
  line L3025 (248.714, 50.3135) -> (249.538, 50.3135) projected
  line L3026 (249.538, 50.3135) -> (249.538, 53.5421) projected
  line L3027 (249.538, 50.3135) -> (249.538, 53.5421) projected
  line L3028 (249.538, 53.5421) -> (256.089, 53.5421) projected
  line L3029 (249.538, 53.5421) -> (256.089, 53.5421) projected
  line L3030 (256.089, 53.5421) -> (256.089, 50.3135) projected
  line L3031 (256.089, 53.5421) -> (256.089, 50.3135) projected
  line L3032 (256.089, 50.3135) -> (257.813, 50.3135) projected
  line L3033 (256.089, 50.3135) -> (257.813, 50.3135) projected
  line L3034 (257.813, 50.3135) -> (257.813, 55.0125) projected
  line L3035 (257.813, 50.3135) -> (257.813, 55.0125) projected
  line L3036 (271.614, 45.9133) -> (271.614, 41.2129) projected
  line L3037 (271.614, 45.9133) -> (271.614, 41.2129) projected
  line L3038 (271.614, 41.2129) -> (257.813, 41.2129) projected
  line L3039 (256.089, 41.4433) -> (254.362, 41.4433) projected
  line L3040 (256.089, 41.4433) -> (254.362, 41.4433) projected
  line L3041 (256.089, 45.9133) -> (256.089, 41.4433) projected
  line L3042 (256.089, 45.9133) -> (256.089, 41.4433) projected
  line L3043 (257.813, 41.2129) -> (257.813, 45.9133) projected
  line L3044 (257.813, 41.2129) -> (257.813, 45.9133) projected
  line L3045 (257.813, 45.9133) -> (256.089, 45.9133) projected
  line L3046 (271.614, 41.2129) -> (257.813, 41.2129) projected
  line L3047 (257.813, 45.9133) -> (256.089, 45.9133) projected
  line L3048 (278.164, 41.4433) -> (278.164, 40.2428) projected
  line L3049 (278.164, 41.4433) -> (278.164, 40.2428) projected
  line L3050 (278.164, 40.2428) -> (275.063, 40.2428) projected
  line L3051 (273.338, 45.9133) -> (271.614, 45.9133) projected
  line L3052 (273.338, 45.9133) -> (271.614, 45.9133) projected
  line L3053 (273.338, 41.4433) -> (273.338, 45.9133) projected
  line L3054 (273.338, 41.4433) -> (273.338, 45.9133) projected
  line L3055 (275.063, 41.4433) -> (273.338, 41.4433) projected
  line L3056 (275.063, 40.2428) -> (275.063, 41.4433) projected
  line L3057 (275.063, 40.2428) -> (275.063, 41.4433) projected
  line L3058 (278.164, 40.2428) -> (275.063, 40.2428) projected
  line L3059 (275.063, 41.4433) -> (273.338, 41.4433) projected
  line L3060 (271.614, 55.0125) -> (271.614, 50.3135) projected
  line L3061 (271.614, 55.0125) -> (271.614, 50.3135) projected
  line L3062 (271.614, 50.3135) -> (273.338, 50.3135) projected
  line L3063 (271.614, 50.3135) -> (273.338, 50.3135) projected
  line L3064 (273.338, 50.3135) -> (273.338, 53.5421) projected
  line L3065 (273.338, 50.3135) -> (273.338, 53.5421) projected
  line L3066 (279.888, 53.5421) -> (279.888, 50.3135) projected
  line L3067 (279.888, 53.5421) -> (279.888, 50.3135) projected
  line L3068 (273.338, 53.5421) -> (279.888, 53.5421) projected
  line L3069 (273.338, 53.5421) -> (279.888, 53.5421) projected
  line L3070 (279.888, 41.4433) -> (278.164, 41.4433) projected
  line L3071 (279.888, 41.4433) -> (278.164, 41.4433) projected
  line L3072 (278.164, 41.4433) -> (278.164, 40.2428) projected
  line L3073 (278.164, 41.4433) -> (278.164, 40.2428) projected
  line L3074 (278.164, 40.2428) -> (275.063, 40.2428) projected
  line L3075 (278.164, 40.2428) -> (275.063, 40.2428) projected
  line L3076 (273.338, 53.5421) -> (279.888, 53.5421) projected
  line L3077 (273.338, 53.5421) -> (279.888, 53.5421) projected
  line L3078 (275.063, 40.2428) -> (275.063, 41.4433) projected
  line L3079 (275.063, 40.2428) -> (275.063, 41.4433) projected
  line L3080 (275.063, 41.4433) -> (273.338, 41.4433) projected
  line L3081 (275.063, 41.4433) -> (273.338, 41.4433) projected
  line L3082 (273.338, 50.3135) -> (273.338, 53.5421) projected
  line L3083 (273.338, 50.3135) -> (273.338, 53.5421) projected
  line L3084 (273.338, 41.4433) -> (273.338, 45.9133) projected
  line L3085 (273.338, 41.4433) -> (273.338, 45.9133) projected
  line L3086 (271.614, 50.3135) -> (273.338, 50.3135) projected
  line L3087 (271.614, 50.3135) -> (273.338, 50.3135) projected
  line L3088 (273.338, 45.9133) -> (271.614, 45.9133) projected
  line L3089 (273.338, 45.9133) -> (271.614, 45.9133) projected
  line L3090 (271.614, 55.0125) -> (271.614, 50.3135) projected
  line L3091 (271.614, 55.0125) -> (271.614, 50.3135) projected
  line L3092 (257.813, 55.0125) -> (271.614, 55.0125) projected
  line L3093 (257.813, 55.0125) -> (271.614, 55.0125) projected
  line L3094 (271.614, 41.2129) -> (257.813, 41.2129) projected
  line L3095 (271.614, 41.2129) -> (257.813, 41.2129) projected
  line L3096 (271.614, 45.9133) -> (271.614, 41.2129) projected
  line L3097 (271.614, 45.9133) -> (271.614, 41.2129) projected
  line L3098 (279.888, 50.3135) -> (280.713, 50.3135) projected
  line L3099 (279.888, 41.4433) -> (278.164, 41.4433) projected
  line L3100 (279.888, 41.4433) -> (278.164, 41.4433) projected
  line L3101 (279.888, 47.7132) -> (279.888, 41.4433) projected
  line L3102 (279.888, 47.7132) -> (279.888, 41.4433) projected
  line L3103 (279.888, 50.3135) -> (280.713, 50.3135) projected
  line L3104 (280.713, 50.3135) -> (280.713, 47.7132) projected
  line L3105 (280.713, 50.3135) -> (280.713, 47.7132) projected
  line L3106 (280.713, 47.7132) -> (279.888, 47.7132) projected
  line L3107 (280.713, 47.7132) -> (279.888, 47.7132) projected
  line L3108 (302.57, 35.9625) -> (302.57, 22.163) projected
  line L3109 (302.57, 35.9625) -> (302.57, 22.163) projected
  line L3110 (302.57, 22.163) -> (288.771, 22.163) projected
  line L3111 (302.57, 22.163) -> (288.771, 22.163) projected
  line L3112 (243.527, 22.163) -> (243.527, 35.9625) projected
  line L3113 (243.527, 22.163) -> (243.527, 35.9625) projected
  line L3114 (250.671, 3.113) -> (250.671, 16.9127) projected
  line L3115 (250.671, 3.113) -> (250.671, 16.9127) projected
  line L3116 (257.327, 22.163) -> (243.527, 22.163) projected
  line L3117 (257.327, 22.163) -> (243.527, 22.163) projected
  line L3118 (243.527, 35.9625) -> (257.327, 35.9625) projected
  line L3119 (243.527, 35.9625) -> (257.327, 35.9625) projected
  line L3120 (257.327, 35.9625) -> (257.327, 22.163) projected
  line L3121 (257.327, 35.9625) -> (257.327, 22.163) projected
  line L3122 (250.671, 16.9127) -> (264.47, 16.9127) projected
  line L3123 (250.671, 16.9127) -> (264.47, 16.9127) projected
  line L3124 (264.47, 3.113) -> (250.671, 3.113) projected
  line L3125 (264.47, 3.113) -> (250.671, 3.113) projected
  line L3126 (264.47, 16.9127) -> (264.47, 3.113) projected
  line L3127 (264.47, 16.9127) -> (264.47, 3.113) projected
  line L3128 (269.721, 22.163) -> (269.721, 35.9625) projected
  line L3129 (269.721, 22.163) -> (269.721, 35.9625) projected
  line L3130 (269.721, 16.9127) -> (283.52, 16.9127) projected
  line L3131 (269.721, 16.9127) -> (283.52, 16.9127) projected
  line L3132 (283.52, 22.163) -> (269.721, 22.163) projected
  line L3133 (283.52, 22.163) -> (269.721, 22.163) projected
  line L3134 (283.52, 3.113) -> (269.721, 3.113) projected
  line L3135 (283.52, 3.113) -> (269.721, 3.113) projected
  line L3136 (283.52, 16.9127) -> (283.52, 3.113) projected
  line L3137 (283.52, 16.9127) -> (283.52, 3.113) projected
  line L3138 (283.52, 35.9625) -> (283.52, 22.163) projected
  line L3139 (283.52, 35.9625) -> (283.52, 22.163) projected
  line L3140 (269.721, 35.9625) -> (283.52, 35.9625) projected
  line L3141 (269.721, 35.9625) -> (283.52, 35.9625) projected
  line L3142 (288.771, 3.113) -> (288.771, 16.9127) projected
  line L3143 (288.771, 3.113) -> (288.771, 16.9127) projected
  line L3144 (288.771, 22.163) -> (288.771, 35.9625) projected
  line L3145 (288.771, 22.163) -> (288.771, 35.9625) projected
  line L3146 (288.771, 35.9625) -> (302.57, 35.9625) projected
  line L3147 (288.771, 35.9625) -> (302.57, 35.9625) projected
  line L3148 (288.771, 16.9127) -> (302.57, 16.9127) projected
  line L3149 (288.771, 16.9127) -> (302.57, 16.9127) projected
  line L3150 (269.721, 3.113) -> (269.721, 16.9127) projected
  line L3151 (269.721, 3.113) -> (269.721, 16.9127) projected
  line L3152 (302.57, 3.113) -> (288.771, 3.113) projected
  line L3153 (302.57, 3.113) -> (288.771, 3.113) projected
  line L3154 (302.57, 16.9127) -> (302.57, 3.113) projected
  line L3155 (302.57, 16.9127) -> (302.57, 3.113) projected
  line L3156 (254.945, 60.2629) -> (241.146, 60.2629) projected
  line L3157 (254.945, 60.2629) -> (241.146, 60.2629) projected
  line L3158 (257.813, 41.2129) -> (257.813, 45.9133) projected
  line L3159 (257.813, 41.2129) -> (257.813, 45.9133) projected
  line L3160 (257.813, 50.3135) -> (257.813, 55.0125) projected
  line L3161 (257.813, 50.3135) -> (257.813, 55.0125) projected
  line L3162 (256.089, 50.3135) -> (257.813, 50.3135) projected
  line L3163 (256.089, 50.3135) -> (257.813, 50.3135) projected
  line L3164 (257.813, 45.9133) -> (256.089, 45.9133) projected
  line L3165 (257.813, 45.9133) -> (256.089, 45.9133) projected
  line L3166 (256.089, 45.9133) -> (256.089, 41.4433) projected
  line L3167 (256.089, 45.9133) -> (256.089, 41.4433) projected
  line L3168 (256.089, 53.5421) -> (256.089, 50.3135) projected
  line L3169 (256.089, 53.5421) -> (256.089, 50.3135) projected
  line L3170 (254.362, 41.4433) -> (254.362, 40.2428) projected
  line L3171 (254.362, 41.4433) -> (254.362, 40.2428) projected
  line L3172 (256.089, 41.4433) -> (254.362, 41.4433) projected
  line L3173 (256.089, 41.4433) -> (254.362, 41.4433) projected
  line L3174 (251.263, 40.2428) -> (251.263, 41.4433) projected
  line L3175 (251.263, 40.2428) -> (251.263, 41.4433) projected
  line L3176 (254.362, 40.2428) -> (251.263, 40.2428) projected
  line L3177 (254.362, 40.2428) -> (251.263, 40.2428) projected
  line L3178 (249.538, 41.4433) -> (249.538, 47.7132) projected
  line L3179 (249.538, 41.4433) -> (249.538, 47.7132) projected
  line L3180 (251.263, 41.4433) -> (249.538, 41.4433) projected
  line L3181 (251.263, 41.4433) -> (249.538, 41.4433) projected
  line L3182 (249.538, 53.5421) -> (256.089, 53.5421) projected
  line L3183 (249.538, 53.5421) -> (256.089, 53.5421) projected
  line L3184 (249.538, 50.3135) -> (249.538, 53.5421) projected
  line L3185 (249.538, 50.3135) -> (249.538, 53.5421) projected
  line L3186 (249.538, 47.7132) -> (248.714, 47.7132) projected
  line L3187 (249.538, 47.7132) -> (248.714, 47.7132) projected
  line L3188 (248.714, 50.3135) -> (249.538, 50.3135) projected
  line L3189 (248.714, 50.3135) -> (249.538, 50.3135) projected
  line L3190 (248.714, 47.7132) -> (248.714, 50.3135) projected
  line L3191 (248.714, 47.7132) -> (248.714, 50.3135) projected
  line L3192 (303.652, 119.844) -> (303.808, 119.826) projected
  line L3193 (303.808, 119.826) -> (303.962, 119.796) projected
  line L3194 (303.962, 119.796) -> (304.115, 119.753) projected
  line L3195 (304.115, 119.753) -> (304.261, 119.698) projected
  line L3196 (304.261, 119.698) -> (304.403, 119.633) projected
  line L3197 (304.403, 119.633) -> (304.541, 119.556) projected
  line L3198 (304.672, 119.469) -> (304.794, 119.371) projected
  line L3199 (304.541, 119.556) -> (304.672, 119.469) projected
  line L3200 (304.794, 119.371) -> (304.91, 119.265) projected
  line L3201 (304.91, 119.265) -> (305.016, 119.149) projected
  line L3202 (305.016, 119.149) -> (305.114, 119.025) projected
  line L3203 (305.114, 119.025) -> (305.201, 118.894) projected
  line L3204 (305.201, 118.894) -> (305.278, 118.758) projected
  line L3205 (305.278, 118.758) -> (305.343, 118.616) projected
  line L3206 (305.343, 118.616) -> (305.398, 118.468) projected
  line L3207 (305.398, 118.468) -> (305.441, 118.317) projected
  line L3208 (305.441, 118.317) -> (305.471, 118.163) projected
  line L3209 (305.471, 1.8741) -> (305.441, 1.7198) projected
  line L3210 (305.398, 1.5696) -> (305.343, 1.4221) projected
  line L3211 (305.343, 1.4221) -> (305.278, 1.2788) projected
  line L3212 (305.278, 1.2788) -> (305.201, 1.1424) projected
  line L3213 (305.201, 1.1424) -> (305.114, 1.0115) projected
  line L3214 (305.441, 1.7198) -> (305.398, 1.5696) projected
  line L3215 (305.114, 1.0115) -> (305.016, 0.8875) projected
  line L3216 (305.016, 0.8875) -> (304.91, 0.7731) projected
  line L3217 (304.794, 0.6656) -> (304.672, 0.5691) projected
  line L3218 (304.672, 0.5691) -> (304.541, 0.4823) projected
  line L3219 (304.541, 0.4823) -> (304.403, 0.4051) projected
  line L3220 (304.91, 0.7731) -> (304.794, 0.6656) projected
  line L3221 (304.403, 0.4051) -> (304.261, 0.339) projected
  line L3222 (304.261, 0.339) -> (304.115, 0.2853) projected
  line L3223 (304.115, 0.2853) -> (303.962, 0.2425) projected
  line L3224 (303.962, 0.2425) -> (303.808, 0.2122) projected
  line L3225 (303.808, 0.2122) -> (303.652, 0.1929) projected
  line L3226 (303.652, 0.1929) -> (303.496, 0.1874) projected
  line L3227 (305.471, 118.163) -> (305.489, 118.007) projected
  line L3228 (305.489, 118.007) -> (305.496, 117.85) projected
  line L3229 (305.496, 117.85) -> (305.496, 2.1869) projected
  line L3230 (305.496, 2.1869) -> (305.489, 2.0298) projected
  line L3231 (305.489, 2.0298) -> (305.471, 1.8741) projected
  line L3232 (2.096, 119.849) -> (303.496, 119.849) projected
  line L3233 (303.496, 0.1874) -> (2.096, 0.1874) projected
  line L3234 (135.883, 116.926) -> (135.883, 103.125) projected
  line L3235 (135.883, 103.125) -> (122.083, 103.125) projected
  line L3236 (122.083, 116.926) -> (135.883, 116.926) projected
  line L3237 (122.083, 103.125) -> (122.083, 116.926) projected
  line L3238 (98.2694, 116.926) -> (112.07, 116.926) projected
  line L3239 (112.07, 103.125) -> (98.2694, 103.125) projected
  line L3240 (112.07, 116.926) -> (112.07, 103.125) projected
  line L3241 (28.7266, 35.9625) -> (14.9269, 35.9625) projected
  line L3242 (23.9641, 55.0125) -> (23.9641, 41.2129) projected
  line L3243 (23.9641, 41.2129) -> (10.163, 41.2129) projected
  line L3244 (10.163, 55.0125) -> (23.9641, 55.0125) projected
  line L3245 (10.163, 41.2129) -> (10.163, 55.0125) projected
  line L3246 (78.0881, 15.4423) -> (78.0881, 12.2136) projected
  line L3247 (78.0881, 12.2136) -> (77.264, 12.2136) projected